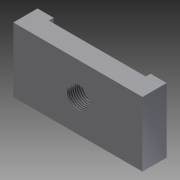
# Autodesk Inventor part: encoder mount
Saved by Autodesk Inventor 2012 (Build 160160000, 160)
## iProperties
Created: 2012-02-02
Part Number: encoder mount
Material: Default
Document SubType Name: Modeling
Designer: caduser
Density: 1 g/cm^3
Author: caduser
Autodesk Inventor part; units mm, degrees
ref_plane "YZ Plane" through (0, 0, 0) normal (1, 0, 0) x (0, 1, 0)
ref_plane "XZ Plane" through (0, 0, 0) normal (0, 1, 0) x (-1, 0, 0)
ref_plane "XY Plane" through (0, 0, 0) normal (0, 0, 1) x (1, 0, 0)
sketch "Sketch1" plane through (0, 0, 0) normal (0, 0, 1) x (1, 0, 0)
  line L0 (-35.56, 0) -> (35.56, 0) projected
  line L1 (0, -20.0025) -> (0, 20.0025) projected
  line L2 (-25.4, 12.7) -> (25.4, 12.7)
  line L3 (25.4, 12.7) -> (25.4, -12.7)
  line L4 (25.4, -12.7) -> (-25.4, -12.7)
  line L5 (-25.4, -12.7) -> (-25.4, 12.7)
  circle A0 centre (0, 0) radius 14.2875 construction
  point P0 (-25.4, 0)
  point P1 (0, 12.7)
  dimension "d0" = 28.575
  dimension "d1" = 50.8
  dimension "d2" = 25.4
  constraints: 8 end point, 2 midpoint, 2 parallel, 1 centre point, 1 coincident, 1 horizontal, 1 horizontal alignment, 1 perpendicular, 1 vertical alignment
  measures "d0" diameter of A0
  measures "d1" distance of L3.end L4.end
  measures "d2" distance of L4.end L2.start
extrude "Extrusion1" add sketch "Sketch1" along normal blind 9.525
sketch "Sketch2" plane through (-25.4, 12.7, 0) normal (0, 1, 0) x (1, 0, 0)
  line L0 (0, -9.525) -> (50.8, -9.525) projected
  line L1 (0, 0) -> (50.8, 0) projected
  line L2 (0, 0) -> (0, -9.525) projected
  line L3 (44.45, 0) -> (44.45, -1.905)
  line L4 (6.35, -1.905) -> (6.35, 0)
  line L5 (6.35, -1.905) -> (44.45, -1.905)
  line L6 (25.4, 0) -> (25.4, -9.525) construction
  dimension "d5" = 6.35
  dimension "d7" = 1.905
  constraints: 8 end point, 2 point on line, 1 midpoint, 1 other
  measures "d5" distance between parallel lines of L2 L4
  measures "d7" distance between parallel lines of L1 L5
extrude "Extrusion2" cut sketch "Sketch2" against normal through all
sketch "Sketch3" plane through (0, 0, 0) normal (0, 0, -1) x (-1, 0, 0)
  line L0 (25.4, 12.7) -> (19.05, 12.7) projected
  line L1 (35.56, 0) -> (-35.56, 0) projected
  line L2 (0, -17.78) -> (0, 17.78) projected
  point P0 (0, 0)
  point P1 (22.225, 7.9375)
  point P2 (22.225, -7.9375)
  point P3 (22.225, 12.7)
  dimension "d10" = 4.7625
  constraints: 1 midpoint, 1 symmetric about line, 1 vertical alignment
  measures "d10" distance from line of L0 point (22.225, 7.938)
hole "Hole1" at (-22.225, 7.9375, 0) at (-22.225, -7.9375, 0) direction (0, 0, 1) diameter 3.683 depth 6.35 tip angle 118 thread size "10-24 UNC" class "2B" standard "ANSI Unified Screw Threads"
mirror "Mirror1" about plane through (0, 0, 0) normal (1, 0, 0) of "Hole1"
sketch "Sketch4" plane through (0, 0, 9.525) normal (0, 0, 1) x (1, 0, 0)
  point P0 (0, 0)
  point P1 (0, 0)
  constraints: 1 coincident
hole "Hole2" at (0, 0, 9.525) direction (0, 0, -1) diameter 8.6614 end through all thread size "3/8-32 UNEF" class "2B" standard "ANSI Unified Screw Threads"
body "Solid1"
